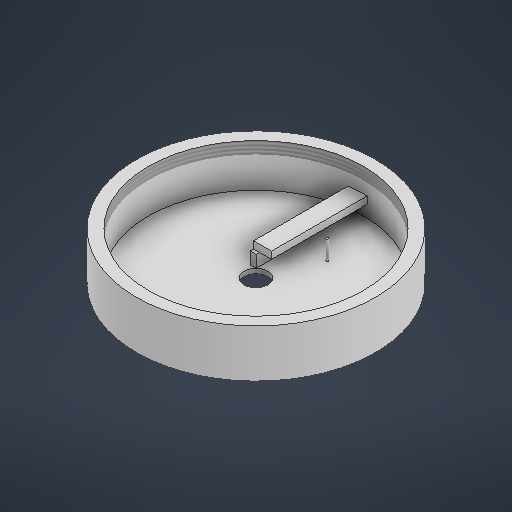
# Autodesk Inventor part: Pieza5
Saved by Autodesk Inventor 2026.1 (Build 301233000, 233)
## iProperties
Created: 2025-09-20
Part Number: Pieza5
Material: Genérico
Document SubType Name: Modeling
Designer: Usuario
Density: 1 g/cm^3
Appearance: Valor por defecto
Author: Usuario
Autodesk Inventor part; units mm, degrees
ref_plane "YZ Plane" through (0, 0, 0) normal (1, 0, 0) x (0, 1, 0)
ref_plane "XZ Plane" through (0, 0, 0) normal (0, 1, 0) x (-1, 0, 0)
ref_plane "XY Plane" through (0, 0, 0) normal (0, 0, 1) x (1, 0, 0)
sketch "Boceto1" plane through (0, 0, 0) normal (0, 1, 0) x (-1, 0, 0)
  circle A0 centre (0, 0) radius 5
  circle A1 centre (0, 0) radius 50
  dimension "d0" = 10
  dimension "d1" = 100
  constraints: 2 centre point, 2 coincident
  measures "d0" diameter of A0
  measures "d1" diameter of A1
extrude "Extrusión1" add sketch "Boceto1" along normal blind 2
sketch "Boceto2" plane through (0, 2, 0) normal (0, 1, 0) x (1, 0, 0)
  circle A0 centre (0, 0) radius 5
  circle A1 centre (0, 0) radius 50
  circle A2 centre (0, 0) radius 45
  line L0 (45, 0) -> (17.222222, 41.573971) construction
  line L1 (17.222222, 41.573971) -> (-3.564763, 27.685082) construction
  line L2 (-3.564763, 27.685082) -> (24.213015, -13.888889) construction
  line L3 (24.213015, -13.888889) -> (45, 0) construction
  line L4 (0, 0) -> (-3.5, 0) construction
  line L5 (-3.5, 0) -> (-3.5, 23.962856) construction
  line L6 (-3.5, 23.962856) -> (0, 23.962856) construction
  line L7 (0, 23.962856) -> (0, 0) construction
  line L8 (0, 0) -> (3.5, 0) construction
  line L9 (3.5, 0) -> (3.5, 23.962856) construction
  line L10 (3.5, 23.962856) -> (0, 23.962856) construction
  line L11 (3.5, 21.339137) -> (8.5, 21.339137) construction
  circle A3 centre (8.5, 21.339137) radius 0.5
  line L12 (-3.5, 3.570714) -> (-3.564763, 44.858583)
  line L13 (-3.564763, 44.858583) -> (-6.06476, 44.854661)
  line L14 (-6.064344, 44.589502) -> (-5.999997, 3.566793)
  line L15 (-5.999997, 3.566793) -> (-3.5, 3.570714)
  dimension "d4" = 100
  dimension "d5" = 90
  dimension "d6" = 50
  dimension "d7" = 25
  dimension "d8" = 3.5
  dimension "d9" = 5
  dimension "d10" = 1
  dimension "d11" = 2.5
  constraints: 32 end point, 5 perpendicular, 4 parallel, 4 point on circle, 3 centre point, 3 coincident, 2 point on line, 2 symmetric about line, 1 horizontal, 2 other
  measures "d4" diameter of A1
  measures "d5" diameter of A2
  measures "d6" distance of L0.start L0.end
  measures "d7" distance of L0.end L1.end
  measures "d8" distance of L4.start L4.end
  measures "d9" distance of L11.start L11.end
  measures "d10" diameter of A3
  measures "d11" distance of L13.end L12.end
sketch "Boceto2 outline for Extrusión2" plane through (0, 2, 0) normal (0, 1, 0) x (1, 0, 0)
  circle A0 centre (8.5, 21.339137) radius 0.5
  circle A1 centre (0, 0) radius 50
  line L0 (-5.999997, 3.566793) -> (-3.5, 3.570714)
  line L1 (-6.064344, 44.589502) -> (-5.999997, 3.566793)
  arc A2 (-3.564763, 44.858583) -> (-6.064344, 44.589502) centre (0, 0) cw
  line L2 (-3.5, 3.570714) -> (-3.564763, 44.858583)
extrude "Extrusión2" add sketch "Boceto2 outline for Extrusión2" along normal blind 5
sketch "Boceto3" plane through (0, 7, 0) normal (0, 1, 0) x (1, 0, 0)
  circle A0 centre (0, 0) radius 5
  circle A1 centre (0, 0) radius 45
  line L0 (-6.064344, 44.589502) -> (-5.999997, 3.566793)
  line L1 (-6.064344, 44.589502) -> (-5.999997, 3.566793)
  line L2 (-5.999997, 3.566793) -> (-3.5, 3.570714)
  line L3 (-3.502248, 5.003921) -> (-3.5, 3.570714)
  line L4 (-6.002245, 5) -> (1.497746, 5.011764)
  line L5 (1.497746, 5.011764) -> (1.497746, 44.975068)
  circle A2 centre (8.5, 21.339137) radius 0.5
  circle A3 centre (8.5, 21.339137) radius 0.5
  circle A4 centre (0, 0) radius 50
  point P0 (-3.564763, 44.858583)
  dimension "d14" = 90
  dimension "d15" = 7.5
  dimension "d16" = 1
  dimension "d17" = 100
  constraints: 10 end point, 3 centre point, 2 coincident, 2 perpendicular, 2 point on circle, 2 point on line, 1 collinear, 1 vertical, 2 other
  measures "d14" diameter of A1
  measures "d15" distance of L4.start L4.end
  measures "d16" diameter of A3
  measures "d17" diameter of A4
sketch "Boceto3 outline for Extrusión3" plane through (0, 7, 0) normal (0, 1, 0) x (1, 0, 0)
  circle A0 centre (8.5, 21.339137) radius 0.5
  circle A1 centre (0, 0) radius 50
  line L0 (1.497746, 5.011764) -> (1.497746, 44.975068)
  line L1 (-6.002245, 5) -> (1.497746, 5.011764)
  line L2 (-6.064344, 44.589502) -> (-6.002245, 5)
  arc A2 (1.497746, 44.975068) -> (-6.064344, 44.589502) centre (0, 0) cw
extrude "Extrusión3" add sketch "Boceto3 outline for Extrusión3" along normal blind 3
sketch "Boceto4" plane through (0, 10, 0) normal (0, 1, 0) x (1, 0, 0)
  circle A0 centre (0, 0) radius 45
  circle A1 centre (0, 0) radius 50
  dimension "d20" = 90
  dimension "d21" = 100
  constraints: 2 centre point, 2 coincident
  measures "d20" diameter of A0
  measures "d21" diameter of A1
extrude "Extrusión4" add sketch "Boceto4" along normal blind 10
thread "Rosca1" size "M75x1.5" class "6H" standard "ANSI Metric M Profile" length 5
